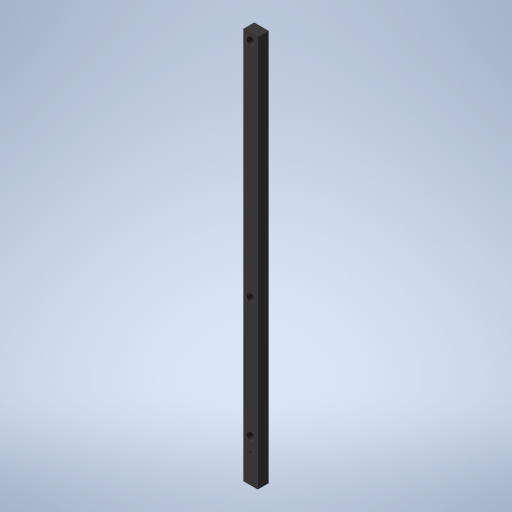
# Autodesk Inventor part: rod(6-32)
Saved by Autodesk Inventor 2024 (Build 280153000, 153)
## iProperties
Created: 2023-04-27
Part Number: rod(6-32)
Material: Generic
Document SubType Name: Modeling
Designer: Fujitsu
Density: 1 g/cm^3
Appearance: Default
Mass: 4.97817 g
Surface Area: 41.5822 cm^2
Volume: 4.97817 cm^3
Author: Fujitsu
Autodesk Inventor part; units mm, degrees
ref_plane "YZ Plane" through (0, 0, 0) normal (1, 0, 0) x (0, 1, 0)
ref_plane "XZ Plane" through (0, 0, 0) normal (0, 1, 0) x (-1, 0, 0)
ref_plane "XY Plane" through (0, 0, 0) normal (0, 0, 1) x (1, 0, 0)
sketch "Sketch1" plane through (0, 0, 0) normal (0, 1, 0) x (-1, 0, 0)
  line L0 (0, 0) -> (6.35, 0)
  line L1 (6.35, 0) -> (6.35, -4.7625)
  line L2 (6.35, -4.7625) -> (0, -4.7625)
  line L3 (0, -4.7625) -> (0, 0)
  circle A0 centre (3.175, -2.3812) radius 1.7526
  dimension "d0" = 6.35
  dimension "d1" = 4.7625
  dimension "d2" = 3.5052
  constraints: 8 end point, 2 parallel, 1 centre point, 1 horizontal, 1 perpendicular
  measures "d0" distance of L1.end L2.end
  measures "d1" distance of L0.end L1.end
  measures "d2" diameter of A0
extrude "Extrusion1" add sketch "Sketch1" along normal blind 176.182 contours L0 L1 L2 L3 | A0
sketch "Sketch2" plane through (-6.35, 0, 0) normal (0, 0, 1) x (1, 0, 0)
  line L0 (6.35, 176.182) -> (0, 176.182) projected
  line L1 (3.175, 176.182) -> (3.175, 173.007)
  circle A0 centre (3.175, 173.007) radius 1.7526
  line L2 (6.35, 0) -> (0, 0) projected
  line L3 (3.175, 0) -> (3.175, 19.05)
  circle A1 centre (3.175, 19.05) radius 1.7526
  line L4 (3.175, 0) -> (3.175, 12.7)
  circle A2 centre (3.175, 12.7) radius 0.508
  line L5 (3.175, 173.007) -> (3.175, 73.007)
  circle A3 centre (3.175, 73.007) radius 1.7526
  dimension "d5" = 3.175
  dimension "d6" = 3.5052
  dimension "d14" = 19.05
  dimension "d15" = 3.5052
  dimension "d16" = 12.7
  dimension "d17" = 1.016
  dimension "d47" = 100.0001
  dimension "d48" = 3.5052
  constraints: 8 end point, 4 centre point, 4 coincident, 3 vertical, 2 midpoint, 1 point on line
  measures "d5" distance of L1.start L1.end
  measures "d6" diameter of A0
  measures "d14" distance of L3.start L3.end
  measures "d15" diameter of A1
  measures "d16" distance of L3.start L4.end
  measures "d17" diameter of A2
  measures "d47" distance of L5.start L5.end
  measures "d48" diameter of A3
hole "Hole2" at (-3.175, 19.05, 0) direction (0, 0, -1) diameter 3.7973 end through all clearance for "Flat Head Machine Screw (82)" size "#6" standard "Ansi Unified Screw Threads"
hole "Hole3" at (-3.175, 12.7, 0) direction (0, 0, -1) diameter 1.016 end through all
hole "Hole4" at (-3.175, 173.007, 0) direction (0, 0, -1) diameter 3.7973 end through all clearance for "Flat Head Machine Screw (82)" size "#6" standard "Ansi Unified Screw Threads"
sketch "Sketch3" plane through (0, 0, 0) normal (0, -1, 0) x (1, 0, 0)
  line L0 (0, -4.7625) -> (-6.35, -4.7625) projected
  line L1 (-6.35, -4.7625) -> (0, 0)
  circle A0 centre (-3.175, -2.3812) radius 1.3208
  dimension "d39" = 2.6416
  constraints: 2 end point, 1 centre point, 1 midpoint
  measures "d39" diameter of A0
hole "Hole5" at (-3.175, 0, -2.3812) direction (0, 1, 0) diameter 3.302 depth 12.7 thread size "8-32 UNC" class "2B" standard "ANSI Unified Screw Threads"
hole "Hole6" at (-3.175, 73.007, 0) direction (0, 0, -1) diameter 3.7973 end through all clearance for "Flat Head Machine Screw (82)" size "#6" standard "Ansi Unified Screw Threads"
body "Solid1"
